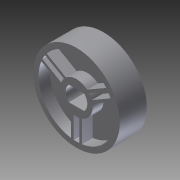
# Autodesk Inventor part: blue wheel hub
Saved by Autodesk Inventor 2012 (Build 160160000, 160)
## iProperties
Created: 2013-10-11
Part Number: blue wheel hub
Material: Default
Document SubType Name: Modeling
Designer: Bryce
Density: 1 g/cm^3
Author: Bryce
Autodesk Inventor part; units mm, degrees
ref_plane "YZ Plane" through (0, 0, 0) normal (1, 0, 0) x (0, 1, 0)
ref_plane "XZ Plane" through (0, 0, 0) normal (0, 1, 0) x (-1, 0, 0)
ref_plane "XY Plane" through (0, 0, 0) normal (0, 0, 1) x (1, 0, 0)
sketch "Sketch1" plane through (0, 0, 0) normal (0, 0, 1) x (1, 0, 0)
  line L0 (-4.4901, 4.4901) -> (4.4901, 4.4901)
  line L1 (4.4901, 4.4901) -> (4.4901, -4.4901) construction
  line L2 (4.4901, -4.4901) -> (-4.4901, -4.4901)
  line L3 (-4.4901, -4.4901) -> (-4.4901, 4.4901) construction
  arc A0 (-4.4901, 4.4901) -> (-4.4901, -4.4901) centre (0, 0) ccw
  arc A1 (4.4901, -4.4901) -> (4.4901, 4.4901) centre (0, 0) ccw
  arc A2 (6.1896, 7.2398) -> (9.3646, 1.7405) centre (0, 0) ccw
  arc A3 (17.4625, 13.7482) -> (20.6375, 8.2489) centre (0, 0) ccw
  circle A4 centre (0, 0) radius 25.4
  line L4 (6.1896, 7.2398) -> (17.4625, 13.7482)
  line L5 (7.3398, 6.0707) -> (18.4045, 12.4589)
  line L6 (19.992, 9.7093) -> (8.9273, 3.3211)
  line L7 (9.3646, 1.7405) -> (20.6375, 8.2489)
  line L8 (0, 0) -> (19.2474, 11.1125) construction
  arc A5 (7.3398, 6.0707) -> (6.1896, 7.2398) centre (0, 0) ccw
  arc A6 (8.9273, 3.3211) -> (7.3398, 6.0707) centre (0, 0) ccw
  arc A7 (9.3646, 1.7405) -> (8.9273, 3.3211) centre (0, 0) ccw
  arc A8 (18.4045, 12.4589) -> (17.4625, 13.7482) centre (0, 0) ccw
  arc A9 (19.992, 9.7093) -> (18.4045, 12.4589) centre (0, 0) ccw
  arc A10 (20.6375, 8.2489) -> (19.992, 9.7093) centre (0, 0) ccw
  line L9 (-9.3646, 1.7405) -> (-20.6375, 8.2489)
  line L10 (-8.9273, 3.3211) -> (-19.992, 9.7093)
  line L11 (-18.4045, 12.4589) -> (-7.3398, 6.0707)
  line L12 (-6.1896, 7.2398) -> (-17.4625, 13.7482)
  arc A11 (-8.9273, 3.3211) -> (-9.3646, 1.7405) centre (0, 0) ccw
  arc A12 (-6.1896, 7.2398) -> (-7.3398, 6.0707) centre (0, 0) ccw
  arc A13 (-19.992, 9.7093) -> (-20.6375, 8.2489) centre (0, 0) ccw
  arc A14 (-17.4625, 13.7482) -> (-18.4045, 12.4589) centre (0, 0) ccw
  line L13 (3.175, -8.9803) -> (3.175, -21.997)
  line L14 (1.5875, -9.3918) -> (1.5875, -22.1682)
  line L15 (-1.5875, -22.1682) -> (-1.5875, -9.3918)
  line L16 (-3.175, -8.9803) -> (-3.175, -21.997)
  arc A15 (1.5875, -9.3918) -> (3.175, -8.9803) centre (0, 0) ccw
  arc A16 (-3.175, -8.9803) -> (-1.5875, -9.3918) centre (0, 0) ccw
  arc A17 (1.5875, -22.1682) -> (3.175, -21.997) centre (0, 0) ccw
  arc A18 (-3.175, -21.997) -> (-1.5875, -22.1682) centre (0, 0) ccw
  dimension "d4" = 6.35
  dimension "d5" = 8.9803
  dimension "d6" = 8.9803
  dimension "d7" = 19.05
  dimension "d8" = 44.45
  dimension "d9" = 50.8
  dimension "d14" = 1.5875
  dimension "d15" = 3.175
  dimension "d16" = 1.5875
  dimension "d17" = 1.5875
  dimension "d18" = 30
  dimension "d21" = 360
  constraints: 40 point on circle, 34 end point, 19 centre point, 7 coincident, 6 parallel, 1 concentric, 1 horizontal, 1 perpendicular, 55 other
  measures "d4" radius of A1
  measures "d5" distance of L0.start L0.end
  measures "d6" distance of L2.end L0.start
  measures "d7" diameter of A2
  measures "d8" diameter of A3
  measures "d9" diameter of A4
  measures "d14" distance between parallel lines of L4 L5
  measures "d15" distance between parallel lines of L6 L5
  measures "d16" distance between parallel lines of L7 L6
  measures "d17" distance between parallel lines of L5 L8
  measures "d18" angle of L8 L0
extrude "Extrusion1" add sketch "Sketch1" along normal mid plane 15.875 contours A5 A6 A7 A2 | L4 A8 L5 A5 | A2 L11 A3 L12 | L6 A10 L7 A7 | A2 L9 A3 L10 | L13 A3 L14 A2 | A2 L15 A3 L16 | A4
extrude "Extrusion2" add sketch "Sketch1" along normal mid plane 3.175 contours A5 A6 A7 A2 | A2 L12 A3 L4 | A2 L11 A3 L12 | L5 A9 L6 A6 | A2 L10 A3 L11 | A2 L9 A3 L10 | L7 A3 L13 A2 | A2 L16 A3 L9 | L13 A3 L14 A2 | A2 L15 A3 L16 | L14 A3 L15 A2
equation "\"d5\" = d6"
equation "\"d16\" = d14"
equation "\"d17\" = 0.5 * d15"
body "Solid1"
